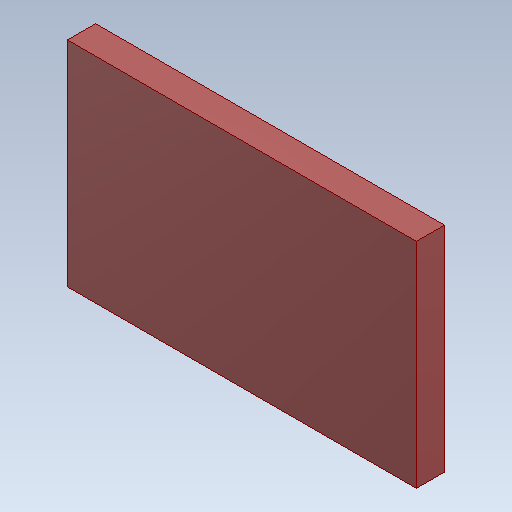
# Autodesk Inventor part: J1_SCREWTERMINAL-5MM-2
Saved by Autodesk Inventor 2020 (Build 240168000, 168)
## iProperties
Created: 2019-08-29
Part Number: J1_SCREWTERMINAL-5MM-2
Material: Generic
Document SubType Name: Modeling
Designer: psrob
Density: 1 g/cm^3
Appearance: SCREWTERMINAL-5MM-2, J1_SCREWTERMINAL-5MM-2
Author: psrob
Autodesk Inventor part; units mm, degrees
ref_plane "YZ Plane" through (0, 0, 0) normal (1, 0, 0) x (0, 1, 0)
ref_plane "XZ Plane" through (0, 0, 0) normal (0, 1, 0) x (-1, 0, 0)
ref_plane "XY Plane" through (0, 0, 0) normal (0, 0, 1) x (1, 0, 0)
sketch "SCREWTERMINAL-5MM-2, J1_SCREWTERMINAL-5MM-2_24" plane through (0, 0, 0) normal (0, 0, 1) x (1, 0, 0)
  line L0 (-3.7, 4.3016) -> (8.7, 4.3016)
  line L1 (8.7, 4.3016) -> (8.7, -3.3)
  line L2 (8.7, -3.3) -> (-3.7, -3.3)
  line L3 (-3.7, -3.3) -> (-3.7, 4.3016)
  constraints: 8 end point
extrude "Extrusion1" add sketch "SCREWTERMINAL-5MM-2, J1_SCREWTERMINAL-5MM-2_24" along normal blind 1
body "Solid1"
